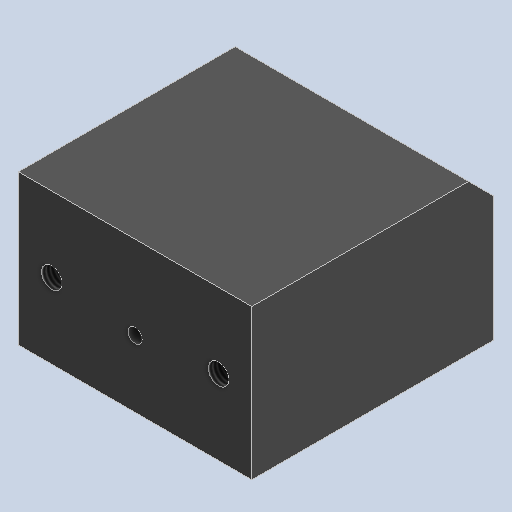
# Autodesk Inventor part: CASE PROT IR
Saved by Autodesk Inventor 2026 (Build 300175050, 175E)
## iProperties
Created: 2025-09-08
Part Number: CASE PROT IR
Material: Poliacetal
Document SubType Name: Modeling
Designer: Kedson Neves
Density: 1.41 g/cm^3
Appearance: Genérico
Author: Kedson Neves
Autodesk Inventor part; units mm, degrees
ref_plane "YZ Plane" through (0, 0, 0) normal (1, 0, 0) x (0, 1, 0)
ref_plane "XZ Plane" through (0, 0, 0) normal (0, 1, 0) x (-1, 0, 0)
ref_plane "XY Plane" through (0, 0, 0) normal (0, 0, 1) x (1, 0, 0)
sketch "Esboço1" plane through (0, 0, 0) normal (0, 0, 1) x (1, 0, 0)
  line L0 (-14, -9) -> (14, -9)
  line L1 (14, -9) -> (14, 9)
  line L2 (14, 9) -> (-14, 9)
  line L3 (-14, 9) -> (-14, -9)
  line L4 (-14, -9) -> (14, 9) construction
  line L5 (14, -9) -> (-14, 9) construction
  point P0 (0, 0)
  dimension "d0" = 18
  dimension "d3" = 28
  constraints: 12 end point, 2 midpoint, 2 parallel, 1 horizontal, 1 perpendicular
  measures "d0" distance of L2.end L0.start
  measures "d3" distance between parallel lines of L1 L3
extrude "Extrusão1" add sketch "Esboço1" along normal blind 29
sketch "Esboço2" plane through (0, 0, 29) normal (0, 0, 1) x (1, 0, 0)
  circle A0 centre (0, -1) radius 0.84
  line L0 (-14, -9) -> (14, -9) projected
  point P0 (0, 0)
  dimension "d4" = 1.68
  dimension "d5" = 8
  constraints: 1 centre point
  measures "d4" diameter of A0
  measures "d5" distance from line of L0 A0.centre
extrude "Extrusão2" cut sketch "Esboço2" against normal blind 20
sketch "Esboço3" plane through (-14, -9, 0) normal (0, -1, 0) x (1, 0, 0)
  line L0 (8, 26.5) -> (20, 26.5)
  line L1 (20, 26.5) -> (20, 3.5)
  line L2 (20, 3.5) -> (8, 3.5)
  line L3 (8, 3.5) -> (8, 26.5)
  line L4 (0, 29) -> (28, 29) projected
  line L5 (0, 0) -> (28, 0) projected
  point P0 (14, 0)
  point P1 (14, 0)
  point P2 (14, 3.5)
  dimension "d8" = 2.5
  dimension "d9" = 12
  dimension "d10" = 0
  dimension "d11" = 23
  constraints: 8 end point, 2 midpoint, 2 parallel, 1 horizontal, 1 perpendicular
  measures "d8" distance between parallel lines of L4 L0
  measures "d9" distance between parallel lines of L1 L3
  measures "d10" horizontal distance of point (14, 0) point (14, 3.5)
  measures "d11" distance between parallel lines of L2 L0
extrude "Extrusão3" cut sketch "Esboço3" against normal blind 12
sketch "Esboço4" plane through (0, 0, 29) normal (0, 0, 1) x (1, 0, 0)
  line L0 (-14, 9) -> (-14, -9) projected
  line L1 (14, -9) -> (14, 9) projected
  point P0 (0, 0)
  point P1 (-10, 0)
  point P2 (10, 0)
  point P3 (-6, -9)
  point P4 (6, -9)
  dimension "d14" = 4
  dimension "d15" = 4
  measures "d14" distance from line of L0 point (-10, 0)
  measures "d15" distance from line of L1 point (10, 0)
hole "Furo1" at (10, 0, 29) at (-10, 0, 29) direction (0, 0, -1) diameter 2.459 depth 16 tip angle 118 thread size "M3x0.5" class "6H" standard "ISO Metric profile"
chamfer "Chanfro1" distance 3 angle 45 1 edges at (0, 9, 0)
fillet "Arredondamento1" radius 1 4 edges at (6, -3, 26.5) (-6, -3, 26.5) (-6, -3, 3.5) (6, -3, 3.5)
